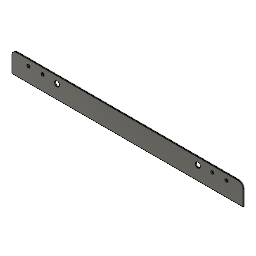
Corsair_1000D_120mm_x_8_FanTray_Ridge_v1 (Autodesk Fusion 360 design; units mm, degrees)
Autodesk Fusion 360 part; units mm, degrees
sketch "Ridge_BIG" plane through (0, 0, 0) normal (0, 1, 0) x (1, 0, 0)
  line L0 (0, 0) -> (244, 0)
  line L1 (244, 0) -> (244, -16.92)
  line L2 (238.92, -22) -> (5.08, -22)
  line L3 (0, -16.92) -> (0, 0)
  circle A0 centre (47.8, -14.5) radius 2.6
  circle A1 centre (196.2, -14.5) radius 2.6
  circle A2 centre (17.7, -15.5) radius 1.5
  circle A3 centre (32.6, -15.5) radius 1.5
  circle A4 centre (211.4104, -15.5) radius 1.5
  circle A5 centre (226.3, -15.5) radius 1.5
  arc A6 (0, -16.92) -> (5.08, -22) centre (5.08, -16.92) ccw
  arc A7 (238.92, -22) -> (244, -16.92) centre (238.92, -16.92) ccw
  point P0 (244, -22)
  dimension "d1" = 244
  dimension "d2" = 22
  dimension "d3" = 5.2
  dimension "d4" = 5.2
  dimension "d5" = 3
  dimension "d6" = 3
  dimension "d7" = 4.9
  dimension "d8" = 45.2
  dimension "d9" = 4.9
  dimension "d10" = 45.2
  dimension "d11" = 31.1
  dimension "d12" = 5
  dimension "d13" = 5
  dimension "d14" = 16.2
  dimension "d15" = 3
  dimension "d16" = 3
  dimension "d17" = 5
  dimension "d18" = 31.0896
  dimension "d20" = 5
  dimension "d21" = 16.2
  dimension "d22" = 5.08
  dimension "d23" = 5.08
  constraint horizontal L0
  constraint vertical L1
  constraint horizontal L2
  constraint vertical L3
  constraint coincident L0.start L3.end
  constraint tangent L3 A6
  constraint tangent L2 A6
  constraint coincident P0 L1
  constraint coincident P0 L2
  constraint tangent L1 A7
  constraint tangent L2 A7
  measures "d1" distance of L0.start L0.end
  measures "d2" distance of L0.end P0
  measures "d3" diameter of A0
  measures "d4" diameter of A1
  measures "d5" diameter of A2
  measures "d6" diameter of A3
  measures "d7" distance of L2 A0 L0.end
  measures "d8" distance of L3 A0
  measures "d9" distance of L2 A1 L0.end
  measures "d10" distance of L1 A1
  measures "d11" distance of L3 A3
  measures "d12" distance of L2 A3 L0.end
  measures "d13" distance of L2 A2 L0.end
  measures "d14" distance of L3 A2
  measures "d15" diameter of A4
  measures "d16" diameter of A5
  measures "d17" distance of L2 A4 L0.end
  measures "d18" distance of L1 A4
  measures "d20" distance of L2 A5 L0.end
  measures "d21" distance of L1 A5
  measures "d22" radius of A6
  measures "d23" radius of A7 L0.end
extrude "Extrude1" add sketch "Ridge_BIG" along normal blind 1.27
